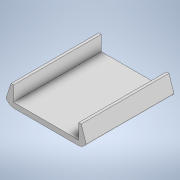
# Autodesk Inventor part: Case_Cover
Saved by Autodesk Inventor 2020 (Build 240168000, 168)
## iProperties
Created: 2019-11-07
Part Number: Case_Cover
Material: 일반
Document SubType Name: Modeling
Designer: Knowblesse
Density: 1 g/cm^3
Appearance: 기본값
Author: Knowblesse
## iProperties of the stored document _3D 인쇄.ipt
Created: 2019-11-07
Part Number: _3D 인쇄
Material: 일반
Document SubType Name: Modeling
Designer: Knowblesse
Density: 1 g/cm^3
Appearance: 기본값
Author: Knowblesse
Autodesk Inventor part; units mm, degrees
ref_plane "YZ Plane" through (0, 0, 0) normal (1, 0, 0) x (0, 1, 0)
ref_plane "XZ Plane" through (0, 0, 0) normal (0, 1, 0) x (-1, 0, 0)
ref_plane "XY Plane" through (0, 0, 0) normal (0, 0, 1) x (1, 0, 0)
sketch "스케치1" plane through (0, 0, 0) normal (0, 1, 0) x (-1, 0, 0)
  line L0 (0, 0) -> (16, 0)
  line L1 (16, 0) -> (16, -17.5)
  line L2 (16, -17.5) -> (0, -17.5)
  line L3 (0, -17.5) -> (0, 0)
  dimension "d0" = 16
  dimension "d1" = 17.5
  constraints: 8 end point, 2 parallel, 1 horizontal, 1 perpendicular
  measures "d0" distance of L1.end L2.end
  measures "d1" distance of L0.end L1.end
extrude "돌출1" add sketch "스케치1" along normal blind 1
sketch "스케치2" plane through (0, 1, 0) normal (0, 1, 0) x (1, 0, 0)
  line L0 (-16, 0) -> (0, 0) projected
  line L1 (0, 0) -> (0, 17.5) projected
  line L2 (0, 17.5) -> (-16, 17.5) projected
  line L3 (-16, 17.5) -> (-16, 0) projected
  line L4 (-16, 0) -> (0, 0) projected
  line L5 (-16, 17.5) -> (-14.5, 17.5)
  line L6 (-14.5, 17.5) -> (-14.5, 0)
  line L7 (-14.5, 0) -> (-16, 0)
  line L8 (-16, 0) -> (-16, 17.5)
  line L9 (0, 17.5) -> (-16, 17.5) projected
  line L10 (0, 0) -> (-1.5, 0)
  line L11 (-1.5, 0) -> (-1.5, 17.5)
  line L12 (-1.5, 17.5) -> (0, 17.5)
  line L13 (0, 17.5) -> (0, 0)
  point P0 (-1.5, 0)
  point P1 (-14.5, 0)
  dimension "d4" = 1.5
  dimension "d5" = 1.5
  constraints: 16 end point, 4 parallel, 2 horizontal, 2 perpendicular, 2 point on line
  measures "d4" distance of L6.end L7.end
  measures "d5" distance of L11.end L12.end
extrude "돌출2" add sketch "스케치2" along normal blind 3 contours L3 L2 L6 L0 | L11 L2 L1 L0
chamfer "모따기1" distance 1 distance2 3 1 edges at (0, 4, -8.75) measured on face at (-0.5, 4, -8.75)
chamfer "모따기2" distance 1 distance2 3 1 edges at (-16, 4, -8.75) measured on face at (-15.5, 4, -8.75)
fillet "모깎기1" radius 2 2 edges at (-16, 0, -8.75) (0, 0, -8.75)
